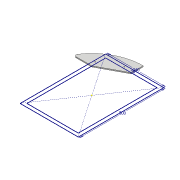
# Autodesk Inventor part: beltMount
Saved by Autodesk Inventor 2018.2 (Build 222227000, 227)
## iProperties
Created: 2018-05-06
Part Number: beltMount
Material: Generic
Document SubType Name: Modeling
Designer: sawaiz
Density: 1 g/cm^3
Appearance: Default
Author: sawaiz
Autodesk Inventor part; units mm, degrees
ref_plane "YZ Plane" through (0, 0, 0) normal (1, 0, 0) x (0, 1, 0)
ref_plane "XZ Plane" through (0, 0, 0) normal (0, 1, 0) x (-1, 0, 0)
ref_plane "XY Plane" through (0, 0, 0) normal (0, 0, 1) x (1, 0, 0)
sketch "Sketch1" plane through (0, 0, 0) normal (0, 0, 1) x (1, 0, 0)
  circle A0 centre (0, 0) radius 300
  dimension "d0" = 600
  constraints: 1 centre point, 1 coincident
  measures "d0" diameter of A0
extrude "Extrusion1" add sketch "Sketch1" along normal blind 6
sketch "Sketch2" plane through (0, 0, 6) normal (0, 0, 1) x (1, 0, 0)
  line L0 (-170, -250) -> (170, -250)
  line L1 (170, -250) -> (170, 250)
  line L2 (170, 250) -> (-170, 250)
  line L3 (-170, 250) -> (-170, -250)
  line L4 (-170, -250) -> (170, 250) construction
  line L5 (170, -250) -> (-170, 250) construction
  line L6 (-150, 230) -> (150, 230)
  line L7 (150, 230) -> (150, -230)
  line L8 (150, -230) -> (-150, -230)
  line L9 (-150, -230) -> (-150, 230)
  point P0 (0, 0)
  dimension "d3" = 340
  dimension "d4" = 500
  dimension "d5" = 20
  constraints: 20 end point, 4 parallel, 2 midpoint, 2 perpendicular, 1 horizontal, 3 other
  measures "d3" distance of L2.end L1.end
  measures "d4" distance of L1.end L0.end
  measures "d5" distance between parallel lines of L2 L6
sketch "Sketch3" plane through (0, 0, 6) normal (0, 0, 1) x (1, 0, 0)
  line L0 (0, 0) -> (-261.0308, 150.7062)
  line L1 (0, 0) -> (261.1835, 150.7944)
  line L2 (0, 0) -> (299.5929, 0) construction
  arc A0 (261.1835, 150.7944) -> (-261.0308, 150.7062) centre (0.1023, -3.0238) ccw
  dimension "d6" = 120
  dimension "d7" = 30
  constraints: 6 end point, 2 point on circle, 1 centre point, 1 horizontal
  measures "d6" angle of L0 L1
  measures "d7" angle of L2 L1
extrude "Extrusion2" cut sketch "Sketch3" along normal through all both and the other way through all keep common part
sketch "Sketch4" plane through (0, 0, 6) normal (0, 0, 1) x (1, 0, 0)
  arc A0 (-20.2802, 299.3137) -> (-259.8076, 150) centre (0, 0) ccw projected
  line L0 (259.8076, 150) -> (0, 0) projected
  line L1 (-259.8076, 150) -> (259.8076, 150)
  line L2 (259.8076, 150) -> (0, 0)
  line L3 (0, 0) -> (-259.8076, 150)
  constraints: 6 end point, 1 collinear, 1 horizontal
extrude "Extrusion3" cut sketch "Sketch4" against normal through all
sketch "Sketch5" plane through (0, 0, 6) normal (0, 0, 1) x (1, 0, 0)
  line L0 (-259.8076, 150) -> (259.8076, 150) projected
  arc A0 (259.8076, 150) -> (0, 300) centre (0, 0) ccw projected
  arc A1 (0, 300) -> (-20.2802, 299.3137) centre (0.1023, -3.0238) ccw projected
  arc A2 (-20.2802, 299.3137) -> (-259.8076, 150) centre (0, 0) ccw projected
  line L1 (-150, 230) -> (150, 230) projected
  line L2 (-150, -230) -> (-150, 230) projected
  line L3 (170, 250) -> (-170, 250) projected
  line L4 (-170, 250) -> (-170, -250) projected
  line L5 (-259.8076, 150) -> (259.8076, 150) projected
  line L6 (-150, 150) -> (0, 230)
  line L7 (0, 300) -> (0, 230)
  constraints: 4 end point, 2 point on line, 1 midpoint, 1 perpendicular
extrude "Extrusion4" cut sketch "Sketch5" against normal through all contours L6 L7 L3 A0 L0 | L3 L7 A0
fillet "Fillet1" radius 10 2 edges at (-259.8076, 150, 3) (-150, 150, 3)
sketch "Sketch6" plane through (0, 0, 6) normal (0, 0, 1) x (1, 0, 0)
  line L0 (0, 230) -> (0, 300) projected
  line L1 (170, 250) -> (-170, 250) projected
  line L2 (-170, 250) -> (-170, -250) projected
  point P0 (0, 0)
  point P1 (-160, 180)
  point P2 (-50, 240)
  dimension "d15" = 50
  dimension "d16" = 70
  dimension "d17" = 10
  dimension "d18" = 10
  measures "d15" distance from line of L0 point (-50, 240)
  measures "d16" distance from line of L1 point (-160, 180)
  measures "d17" distance from line of L1 point (-50, 240)
  measures "d18" distance from line of L2 point (-160, 180)
hole "Hole1" at (-160, 180, 6) at (-50, 240, 6) direction (0, 0, -1) diameter 5 end through all
body "Solid1"
